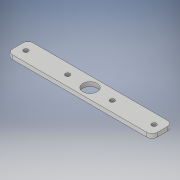
# Autodesk Inventor part: Main Rod v1
Saved by Autodesk Inventor 2018 (Build 220112000, 112)
## iProperties
Created: 2019-12-10
Part Number: Main Rod v1
Material: Generic
Document SubType Name: Modeling
Designer: AOFUser
Density: 1 g/cm^3
Appearance: Default
Author: AOFUser
Autodesk Inventor part; units mm, degrees
ref_plane "YZ Plane" through (0, 0, 0) normal (1, 0, 0) x (0, 1, 0)
ref_plane "XZ Plane" through (0, 0, 0) normal (0, 1, 0) x (-1, 0, 0)
ref_plane "XY Plane" through (0, 0, 0) normal (0, 0, 1) x (1, 0, 0)
sketch "Sketch1" plane through (0, 0, 0) normal (0, 1, 0) x (-1, 0, 0)
  line L0 (0, 0) -> (-88.9, 0)
  line L1 (-88.9, 0) -> (-88.9, -12.7)
  line L2 (-88.9, -12.7) -> (0, -12.7)
  line L3 (0, -12.7) -> (0, 0)
  dimension "d0" = 88.9
  dimension "d1" = 12.7
  constraints: 8 end point, 2 parallel, 1 horizontal, 1 perpendicular
  measures "d0" distance of L2.end L1.end
  measures "d1" distance of L1.end L0.end
extrude "Extrusion1" add sketch "Sketch1" along normal blind 2.54
fillet "Fillet1" radius 3.175 4 edges at (88.9, 1.27, 0) (88.9, 1.27, -12.7) (0, 1.27, -12.7) (0, 1.27, 0)
sketch "Sketch2" plane through (0, 2.54, 0) normal (0, 1, 0) x (1, 0, 0)
  line L0 (88.9, 3.175) -> (88.9, 9.525) projected
  line L1 (88.9, 6.35) -> (44.45, 6.35)
  circle A0 centre (44.45, 6.35) radius 4.445
  point P0 (0, 0)
  dimension "d5" = 44.45
  dimension "d6" = 8.89
  constraints: 2 end point, 1 centre point, 1 coincident, 1 horizontal, 1 midpoint
  measures "d5" distance of L1.start L1.end
  measures "d6" diameter of A0
extrude "Extrusion2" cut sketch "Sketch2" against normal blind 2.54
sketch "Sketch3" plane through (0, 2.54, 0) normal (0, 1, 0) x (1, 0, 0)
  line L0 (3.175, 0) -> (85.725, 0) projected
  line L1 (44.45, 0) -> (44.45, 12.7)
  line L2 (85.725, 12.7) -> (3.175, 12.7) projected
  line L3 (44.45, 6.35) -> (58.166, 6.35)
  point P0 (0, 0)
  dimension "d9" = 13.716
  constraints: 4 end point, 3 midpoint, 1 horizontal
  measures "d9" distance of L3.start L3.end
hole "Hole1" at (58.166, 2.54, -6.35) direction (0, -1, 0) diameter 2.794 end through all
sketch "Sketch4" plane through (0, 2.54, 0) normal (0, 1, 0) x (1, 0, 0)
  line L0 (85.725, 12.7) -> (3.175, 12.7) projected
  line L1 (44.45, 12.7) -> (44.45, 0)
  line L2 (3.175, 0) -> (85.725, 0) projected
  line L3 (44.45, 6.35) -> (30.734, 6.35)
  point P0 (0, 0)
  dimension "d17" = 13.716
  constraints: 4 end point, 3 midpoint, 1 horizontal
  measures "d17" distance of L3.start L3.end
hole "Hole2" at (30.734, 2.54, -6.35) direction (0, -1, 0) diameter 2.794 end through all
sketch "Sketch5" plane through (0, 2.54, 0) normal (0, 1, 0) x (1, 0, 0)
  line L0 (0, 9.525) -> (0, 3.175) projected
  line L1 (0, 6.35) -> (5.08, 6.35)
  point P0 (0, 0)
  dimension "d25" = 5.08
  constraints: 2 end point, 1 horizontal, 1 midpoint
  measures "d25" distance of L1.start L1.end
hole "Hole3" at (5.08, 2.54, -6.35) direction (0, -1, 0) diameter 2.794 end through all
sketch "Sketch6" plane through (0, 2.54, 0) normal (0, 1, 0) x (1, 0, 0)
  line L0 (88.9, 3.175) -> (88.9, 9.525) projected
  line L1 (88.9, 6.35) -> (83.82, 6.35)
  point P0 (0, 0)
  dimension "d33" = 5.08
  constraints: 2 end point, 1 horizontal, 1 midpoint
  measures "d33" distance of L1.start L1.end
hole "Hole4" at (83.82, 2.54, -6.35) direction (0, -1, 0) diameter 2.794 end through all
body "Solid1"
